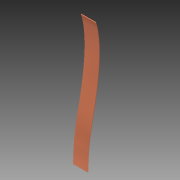
# Autodesk Inventor part: FPCB_1
Saved by Autodesk Inventor 2011 SP2 (Build 150309200, 309)
## iProperties
Created: 2012-02-24
Part Number: FPCB_1
Document SubType Name: Modeling
Designer: sungwook
Density: 1 g/cm^3
Author: sungwook
Autodesk Inventor part; units mm, degrees
ref_plane "YZ Plane" through (0, 0, 0) normal (1, 0, 0) x (0, 1, 0)
ref_plane "XZ Plane" through (0, 0, 0) normal (0, 1, 0) x (-1, 0, 0)
ref_plane "XY Plane" through (0, 0, 0) normal (0, 0, 1) x (1, 0, 0)
sketch "Sketch1" plane through (0, 0, 0) normal (0, 0, 1) x (1, 0, 0)
  line L0 (-1.75, -6.35) -> (1.75, -6.35)
  line L1 (1.75, -6.35) -> (1.75, -6.47)
  line L2 (1.75, -6.47) -> (-1.75, -6.47)
  line L3 (-1.75, -6.47) -> (-1.75, -6.35)
  point P0 (0, 0)
  point P1 (0, -6.35)
  point P2 (-1.75, -6.41)
  dimension "d0" = 3.5
  dimension "d1" = 0.12
  dimension "d4" = 6.35
  constraints: 8 end point, 2 midpoint, 2 parallel, 1 horizontal, 1 perpendicular, 1 vertical alignment
  measures "d0" distance of L0.end L0.start
  measures "d1" distance of L1.end L0.end
  measures "d4" distance of point (0, -6.35) point (0, 0)
sketch "Sketch2" plane through (0, 0, 0) normal (1, 0, 0) x (0, 1, 0)
  line L0 (0, -6.4997) -> (0, 36.4341) projected
  spline S0 degree 4 poles (-4.4704, 30) (-1.8786, 21.8549) (-5.4695, 8.9345) (-6.1177, 8.8786) (-6.35, 0) knots 0 0 0 0 0 1 1 1 1 1
  point P0 (0, 0)
  point P1 (-6.47, 0)
  point P2 (-3.8211, 19.0942)
  point P3 (-5.9065, 6.368)
  point P4 (-5.055, 11.1843)
  dimension "d2" = 4.4704
  dimension "d3" = 30
  constraints: 5 other
  measures "d2" distance from line of L0 point (-4.47, 30)
  measures "d3" vertical distance of point (0, 0) point (-4.47, 30)
sweep "Sweep1" add profiles "Sketch1" path "Sketch2" path curves S0
body "Solid1"
